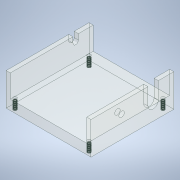
# Autodesk Inventor part: U-shape_v3_0
Saved by Autodesk Inventor 2020 (Build 240168000, 168)
## iProperties
Created: 2022-08-05
Part Number: U-shape_v3_0
Material: Glass
Document SubType Name: Modeling
Designer: Administrator
Density: 2.18 g/cm^3
Appearance: Clear
Author: Administrator
Autodesk Inventor part; units mm, degrees
ref_plane "YZ Plane" through (0, 0, 0) normal (1, 0, 0) x (0, 1, 0)
ref_plane "XZ Plane" through (0, 0, 0) normal (0, 1, 0) x (-1, 0, 0)
ref_plane "XY Plane" through (0, 0, 0) normal (0, 0, 1) x (1, 0, 0)
sketch "Sketch1" plane through (0, 0, 0) normal (0, 1, 0) x (-1, 0, 0)
  line L0 (-43, 37) -> (43, 37)
  line L1 (43, 37) -> (43, -37)
  line L2 (43, -37) -> (-43, -37)
  line L3 (-43, -37) -> (-43, 37)
  line L4 (-43, 37) -> (43, -37) construction
  line L5 (43, 37) -> (-43, -37) construction
  point P0 (0, 0)
  dimension "d0" = 86
  dimension "d1" = 74
  constraints: 12 end point, 2 midpoint, 2 parallel, 1 horizontal, 1 perpendicular
  measures "d0" distance of L1.end L2.end
  measures "d1" distance of L0.end L1.end
extrude "Extrusion1" add sketch "Sketch1" along normal blind 33
sketch "Sketch2" plane through (0, 33, 0) normal (0, 1, 0) x (1, 0, 0)
  line L0 (-43, -37) -> (43, -37) projected
  line L1 (38.75, 40) -> (-38.75, 40)
  line L2 (-38.75, 40) -> (-38.75, -40)
  line L3 (-38.75, -40) -> (38.75, -40)
  line L4 (38.75, -40) -> (38.75, 40)
  line L5 (-38.75, 40) -> (38.75, -40)
  line L6 (-38.75, -40) -> (38.75, 40)
  line L7 (0, 0) -> (-3.3933, 0)
  point P0 (38.75, -37)
  point P1 (-38.75, -37)
  dimension "d8" = 77.5
  dimension "d45" = 80
  constraints: 14 end point, 2 horizontal, 2 parallel, 1 midpoint, 1 perpendicular
  measures "d8" distance of L3.end L2.end
  measures "d45" distance of L3.end L1.start
extrude "Extrusion2" cut sketch "Sketch2" against normal blind 23
sketch "Sketch4" plane through (43, 0, 37) normal (1, 0, 0) x (0, 0, -1)
  line L0 (0, 0) -> (53, 0)
  line L1 (0, 0) -> (74, 0) projected
  line L2 (0, 33) -> (74, 33) projected
  arc A0 (47.75, 16) -> (58.25, 16) centre (53, 16) ccw
  line L3 (58.25, 16) -> (58.25, 33)
  line L4 (74, 33) -> (0, 33) projected
  line L5 (47.75, 16) -> (47.75, 33)
  line L6 (47.75, 33) -> (21.05, 33)
  line L7 (74, 33) -> (0, 33) projected
  line L8 (21.05, 33) -> (21.05, 22.1)
  circle A1 centre (21.05, 22.1) radius 2.75
  point P0 (37, 0)
  dimension "d9" = 53
  dimension "d12" = 10.5
  dimension "d13" = 16
  dimension "d42" = 26.7
  dimension "d43" = 10.9
  dimension "d44" = 5.5
  constraints: 10 end point, 4 point on line, 2 centre point, 2 perpendicular, 2 point on circle, 1 coincident, 1 tangent, 1 vertical
  measures "d9" distance of L0.start L0.end
  measures "d12" diameter of A0
  measures "d13" distance from line of L0 A0.centre
  measures "d42" distance of L5.end L6.end
  measures "d43" distance of L6.end L8.end
  measures "d44" diameter of A1
extrude "Extrusion3" cut sketch "Sketch4" against normal blind 5
sketch "Sketch6" plane through (-43, 0, 37) normal (0, 0, 1) x (1, 0, 0)
  line L0 (86, 0) -> (0, 0) projected
  line L1 (0, 33) -> (86, 33) projected
  line L2 (86, 0) -> (86, 33)
  line L3 (86, 33) -> (81.75, 33)
  line L4 (81.75, 33) -> (81.75, 10)
  line L5 (4.25, 33) -> (4.25, 10) projected
  line L6 (81.75, 10) -> (4.25, 10)
  line L7 (4.25, 10) -> (4.25, 33)
  line L8 (0, 0) -> (0, 33) projected
  line L9 (4.25, 33) -> (0, 33)
  line L10 (0, 33) -> (0, 0)
  line L11 (0, 0) -> (86, 0)
  point P0 (43, 0)
  point P1 (77.5, 2)
  constraints: 16 end point, 7 perpendicular, 1 vertical
extrude "Extrusion4" add sketch "Sketch6" along normal blind 10 contours L0 L8 L1 L5 L6 L4 L2
sketch "Sketch7" plane through (0, 0, 0) normal (0, -1, 0) x (1, 0, 0)
  line L0 (-37.5, -31.5) -> (37.5, -31.5)
  line L1 (37.5, -31.5) -> (37.5, 43.5)
  line L2 (37.5, 43.5) -> (-37.5, 43.5)
  line L3 (-37.5, 43.5) -> (-37.5, -31.5)
  line L4 (-37.5, -31.5) -> (37.5, 43.5) construction
  line L5 (37.5, -31.5) -> (-37.5, 43.5) construction
  circle A0 centre (37.5, 43.5) radius 1.675
  circle A1 centre (37.5, -31.5) radius 1.675
  circle A2 centre (-37.5, 43.5) radius 1.675
  circle A3 centre (-37.5, -31.5) radius 1.675
  point P0 (0, 0)
  dimension "d20" = 75
  dimension "d21" = 75
  dimension "d23" = 3.35
  dimension "d26" = 75
  dimension "d29" = 75
  constraints: 12 end point, 4 centre point, 2 horizontal, 2 parallel, 1 coincident, 1 perpendicular, 1 vertical, 6 other
  measures "d20" distance of L2.end L1.end
  measures "d21" distance of L1.end L0.end
  measures "d23" diameter of A0
  measures "d26" distance of A0.centre A1.centre
  measures "d29" distance of A0.centre A2.centre
extrude "Extrusion5" cut sketch "Sketch7" against normal blind 10 contours L3 A3 L0 | L0 A3 L3 | A1 L1 L0 | L0 L1 A1 | A2 L2 L3 | L3 L2 A2 | A0 L2 L1 | L1 L2 A0
thread "Thread1" size "M3x0.5" class "6H" standard "ANSI Metric M Profile" full length
thread "Thread2" size "M3x0.5" class "6H" standard "ANSI Metric M Profile" full length
thread "Thread3" size "M3x0.5" class "6H" standard "ANSI Metric M Profile" full length
thread "Thread4" size "M3x0.5" class "6H" standard "ANSI Metric M Profile" full length
sketch "Sketch8" plane through (-43, 0, -37) normal (-1, 0, 0) x (0, 0, 1)
  line L0 (84, 10) -> (0, 10) projected
  line L1 (15.75, 10) -> (15.75, 0)
  line L2 (0, 0) -> (84, 0) projected
  line L3 (15.75, 0) -> (17.75, 0)
  line L4 (17.75, 0) -> (17.75, 27.4)
  circle A0 centre (17.75, 27.4) radius 2.75
  line L5 (15.75, 33) -> (15.75, 16) projected
  line L6 (20.5, 27.4) -> (20.5, 33)
  line L7 (15, 27.4) -> (15, 33)
  line L8 (0, 33) -> (84, 33) projected
  point P0 (37, 0)
  point P1 (17.228, 33)
  point P2 (18.272, 33)
  dimension "d46" = 2
  dimension "d47" = 27.4
  dimension "d48" = 5.5
  dimension "d51" = 0
  constraints: 10 end point, 5 point on line, 3 vertical, 2 point on circle, 1 centre point, 1 coincident, 1 perpendicular, 1 tangent
  measures "d46" distance of L1.end L3.end
  measures "d47" distance of L3.end L4.end
  measures "d48" diameter of A0
  measures "d51" distance from line of L5 L1.end
extrude "Extrusion6" cut sketch "Sketch8" against normal blind 10 contours A0 L5 | A0 L5 | A0 L5 L8 L6 | L7 L8 L5 A0
sketch "Sketch10" plane through (37.5, 8, 43.5) normal (1, 0, 0) x (0, 0, 1)
  line L0 (1.675, 0) -> (1.675, 8)
  line L1 (1.675, 8) -> (1.3043, 8)
  line L2 (1.3043, 8) -> (1.3043, 0)
  line L3 (1.3043, 0) -> (1.675, 0)
  line L4 (0, -1.6) -> (0, 9.6) projected
  constraints: 8 end point
revolve "Revolution1" add sketch "Sketch10" angle 360 about axis through (37.5, 8, 43.5) along (0, -1, 0) separate body
sketch "Sketch9" plane through (37.5, 8, 45.175) normal (-1, 0, 0) x (0, -1, 0)
  line L0 (-0.2918, -0.0255) -> (-0.2501, -0.0255) construction
  line L1 (0.0416, -0.3456) -> (-0.0001, -0.4257) construction
  line L2 (-0.5001, -0.4257) -> (-0.5418, -0.3456) construction
  line L3 (-0.2084, -0.0255) -> (-0.2501, 0.0546) construction
  line L4 (-0.2501, 0.0546) -> (-0.2918, -0.0255) construction
  line L5 (-0.5001, -0.4257) -> (-0.4584, -0.3456) construction
  line L6 (-0.2084, -0.0255) -> (-0.0418, -0.3456)
  line L7 (-0.5418, -0.3456) -> (-0.4584, -0.3456) construction
  arc A0 (-0.5418, -0.3456) -> (-0.5001, -0.3709) centre (-0.5001, -0.3239) ccw construction
  line L8 (0.0416, -0.3456) -> (-0.0418, -0.3456) construction
  line L9 (-0.5001, -0.4257) -> (-0.5001, -0.3456) construction
  line L10 (-0.0001, -0.4257) -> (-0.0001, -0.3456) construction
  line L11 (-0.2501, 0.0546) -> (-0.2501, -0.0002) construction
  line L12 (-0.5001, -0.3709) -> (-0.0001, -0.3709)
  arc A1 (-0.5001, -0.3709) -> (-0.4584, -0.3456) centre (-0.5001, -0.3239) ccw
  line L13 (-0.0418, -0.3456) -> (-0.0001, -0.4257) construction
  line L14 (-0.4584, -0.3456) -> (-0.2918, -0.0255)
  line L15 (-0.0001, -0.0002) -> (-0.0001, 0.0177)
  line L16 (-0.0001, 0.0177) -> (-0.0001, -0.0002)
  line L17 (-0.0001, -0.0002) -> (0.0334, -0.0002)
  arc A2 (-0.0418, -0.3456) -> (-0.0001, -0.3709) centre (-0.0001, -0.3239) ccw
  arc A3 (-0.0001, -0.3709) -> (0.0416, -0.3456) centre (-0.0001, -0.3239) ccw construction
  arc A4 (-0.2501, -0.0002) -> (-0.2918, -0.0255) centre (-0.2501, -0.0471) ccw
  arc A5 (-0.2084, -0.0255) -> (-0.2501, -0.0002) centre (-0.2501, -0.0471) ccw
  line L18 (-0.2501, -0.0002) -> (-0.2501, -0.0255) construction
  line L19 (-0.2501, -0.0255) -> (-0.2084, -0.0255) construction
  dimension "d52" = 55
  dimension "d53" = 0.08
  dimension "d54" = 0.08
  dimension "Sketch9_ThreadOffset" = 0
  dimension "Sketch9_MajorRadius" = 0.3707
  dimension "d57" = 0.5
  dimension "Sketch9_MinorRadius" = 0
  constraints: 40 end point, 12 point on circle, 10 parallel, 8 tangent, 6 centre point, 6 collinear, 2 midpoint, 2 point on line, 1 horizontal, 1 perpendicular, 3 other
  measures "d52" angle of L6 L14
  measures "d53" distance of L3.end L0.end
  measures "d54" distance of L1.end L10.end
  measures "Sketch9_ThreadOffset" distance between parallel lines of L15 L10
  measures "Sketch9_MajorRadius" distance from line of L12 L15.start
  measures "d57" distance from line of L1.end L9
  measures "Sketch9_MinorRadius" distance edge to line of A5 L17
coil "Coil1" sketch "Sketch9" operation cut axis through (37.5, 8, 43.5) along (0, -1, 0) pitch 0.5005 turns 17.982018 hand right bodies 2
sketch "Sketch12" plane through (-37.5, 8, 43.5) normal (1, 0, 0) x (0, 0, 1)
  line L0 (1.675, 0) -> (1.675, 8)
  line L1 (1.675, 8) -> (1.3043, 8)
  line L2 (1.3043, 8) -> (1.3043, 0)
  line L3 (1.3043, 0) -> (1.675, 0)
  line L4 (0, -1.6) -> (0, 9.6) projected
  constraints: 8 end point
revolve "Revolution2" add sketch "Sketch12" angle 360 about axis through (-37.5, 8, 43.5) along (0, -1, 0) separate body
sketch "Sketch11" plane through (-37.5, 8, 45.175) normal (-1, 0, 0) x (0, -1, 0)
  line L0 (-0.2918, -0.0255) -> (-0.2501, -0.0255) construction
  line L1 (0.0416, -0.3456) -> (-0.0001, -0.4257) construction
  line L2 (-0.5001, -0.4257) -> (-0.5418, -0.3456) construction
  line L3 (-0.2084, -0.0255) -> (-0.2501, 0.0546) construction
  line L4 (-0.2501, 0.0546) -> (-0.2918, -0.0255) construction
  line L5 (-0.5001, -0.4257) -> (-0.4584, -0.3456) construction
  line L6 (-0.2084, -0.0255) -> (-0.0418, -0.3456)
  line L7 (-0.5418, -0.3456) -> (-0.4584, -0.3456) construction
  arc A0 (-0.5418, -0.3456) -> (-0.5001, -0.3709) centre (-0.5001, -0.3239) ccw construction
  line L8 (0.0416, -0.3456) -> (-0.0418, -0.3456) construction
  line L9 (-0.5001, -0.4257) -> (-0.5001, -0.3456) construction
  line L10 (-0.0001, -0.4257) -> (-0.0001, -0.3456) construction
  line L11 (-0.2501, 0.0546) -> (-0.2501, -0.0002) construction
  line L12 (-0.5001, -0.3709) -> (-0.0001, -0.3709)
  arc A1 (-0.5001, -0.3709) -> (-0.4584, -0.3456) centre (-0.5001, -0.3239) ccw
  line L13 (-0.0418, -0.3456) -> (-0.0001, -0.4257) construction
  line L14 (-0.4584, -0.3456) -> (-0.2918, -0.0255)
  line L15 (-0.0001, -0.0002) -> (-0.0001, 0.0177)
  line L16 (-0.0001, 0.0177) -> (-0.0001, -0.0002)
  line L17 (-0.0001, -0.0002) -> (0.0334, -0.0002)
  arc A2 (-0.0418, -0.3456) -> (-0.0001, -0.3709) centre (-0.0001, -0.3239) ccw
  arc A3 (-0.0001, -0.3709) -> (0.0416, -0.3456) centre (-0.0001, -0.3239) ccw construction
  arc A4 (-0.2501, -0.0002) -> (-0.2918, -0.0255) centre (-0.2501, -0.0471) ccw
  arc A5 (-0.2084, -0.0255) -> (-0.2501, -0.0002) centre (-0.2501, -0.0471) ccw
  line L18 (-0.2501, -0.0002) -> (-0.2501, -0.0255) construction
  line L19 (-0.2501, -0.0255) -> (-0.2084, -0.0255) construction
  dimension "d70" = 55
  dimension "d71" = 0.08
  dimension "d72" = 0.08
  dimension "Sketch11_ThreadOffset" = 0
  dimension "Sketch11_MajorRadius" = 0.3707
  dimension "d75" = 0.5
  dimension "Sketch11_MinorRadius" = 0
  constraints: 40 end point, 12 point on circle, 10 parallel, 8 tangent, 6 centre point, 6 collinear, 2 midpoint, 2 point on line, 1 horizontal, 1 perpendicular, 3 other
  measures "d70" angle of L6 L14
  measures "d71" distance of L3.end L0.end
  measures "d72" distance of L1.end L10.end
  measures "Sketch11_ThreadOffset" distance between parallel lines of L15 L10
  measures "Sketch11_MajorRadius" distance from line of L12 L15.start
  measures "d75" distance from line of L1.end L9
  measures "Sketch11_MinorRadius" distance edge to line of A5 L17
coil "Coil2" sketch "Sketch11" operation cut axis through (-37.5, 8, 43.5) along (0, -1, 0) pitch 0.5005 turns 17.982018 hand right bodies 3
sketch "Sketch14" plane through (37.5, 8, -31.5) normal (1, 0, 0) x (0, 0, 1)
  line L0 (1.675, 0) -> (1.675, 8)
  line L1 (1.675, 8) -> (1.3043, 8)
  line L2 (1.3043, 8) -> (1.3043, 0)
  line L3 (1.3043, 0) -> (1.675, 0)
  line L4 (0, -1.6) -> (0, 9.6) projected
  constraints: 8 end point
revolve "Revolution3" add sketch "Sketch14" angle 360 about axis through (37.5, 8, -31.5) along (0, -1, 0) separate body
sketch "Sketch13" plane through (37.5, 8, -29.825) normal (-1, 0, 0) x (0, -1, 0)
  line L0 (-0.2918, -0.0255) -> (-0.2501, -0.0255) construction
  line L1 (0.0416, -0.3456) -> (-0.0001, -0.4257) construction
  line L2 (-0.5001, -0.4257) -> (-0.5418, -0.3456) construction
  line L3 (-0.2084, -0.0255) -> (-0.2501, 0.0546) construction
  line L4 (-0.2501, 0.0546) -> (-0.2918, -0.0255) construction
  line L5 (-0.5001, -0.4257) -> (-0.4584, -0.3456) construction
  line L6 (-0.2084, -0.0255) -> (-0.0418, -0.3456)
  line L7 (-0.5418, -0.3456) -> (-0.4584, -0.3456) construction
  arc A0 (-0.5418, -0.3456) -> (-0.5001, -0.3709) centre (-0.5001, -0.3239) ccw construction
  line L8 (0.0416, -0.3456) -> (-0.0418, -0.3456) construction
  line L9 (-0.5001, -0.4257) -> (-0.5001, -0.3456) construction
  line L10 (-0.0001, -0.4257) -> (-0.0001, -0.3456) construction
  line L11 (-0.2501, 0.0546) -> (-0.2501, -0.0002) construction
  line L12 (-0.5001, -0.3709) -> (-0.0001, -0.3709)
  arc A1 (-0.5001, -0.3709) -> (-0.4584, -0.3456) centre (-0.5001, -0.3239) ccw
  line L13 (-0.0418, -0.3456) -> (-0.0001, -0.4257) construction
  line L14 (-0.4584, -0.3456) -> (-0.2918, -0.0255)
  line L15 (-0.0001, -0.0002) -> (-0.0001, 0.0177)
  line L16 (-0.0001, 0.0177) -> (-0.0001, -0.0002)
  line L17 (-0.0001, -0.0002) -> (0.0334, -0.0002)
  arc A2 (-0.0418, -0.3456) -> (-0.0001, -0.3709) centre (-0.0001, -0.3239) ccw
  arc A3 (-0.0001, -0.3709) -> (0.0416, -0.3456) centre (-0.0001, -0.3239) ccw construction
  arc A4 (-0.2501, -0.0002) -> (-0.2918, -0.0255) centre (-0.2501, -0.0471) ccw
  arc A5 (-0.2084, -0.0255) -> (-0.2501, -0.0002) centre (-0.2501, -0.0471) ccw
  line L18 (-0.2501, -0.0002) -> (-0.2501, -0.0255) construction
  line L19 (-0.2501, -0.0255) -> (-0.2084, -0.0255) construction
  dimension "d88" = 55
  dimension "d89" = 0.08
  dimension "d90" = 0.08
  dimension "Sketch13_ThreadOffset" = 0
  dimension "Sketch13_MajorRadius" = 0.3707
  dimension "d93" = 0.5
  dimension "Sketch13_MinorRadius" = 0
  constraints: 40 end point, 12 point on circle, 10 parallel, 8 tangent, 6 centre point, 6 collinear, 2 midpoint, 2 point on line, 1 horizontal, 1 perpendicular, 3 other
  measures "d88" angle of L6 L14
  measures "d89" distance of L3.end L0.end
  measures "d90" distance of L1.end L10.end
  measures "Sketch13_ThreadOffset" distance between parallel lines of L15 L10
  measures "Sketch13_MajorRadius" distance from line of L12 L15.start
  measures "d93" distance from line of L1.end L9
  measures "Sketch13_MinorRadius" distance edge to line of A5 L17
coil "Coil3" sketch "Sketch13" operation cut axis through (37.5, 8, -31.5) along (0, -1, 0) pitch 0.5005 turns 17.982018 hand right bodies 4
sketch "Sketch16" plane through (-37.5, 8, -31.5) normal (1, 0, 0) x (0, 0, 1)
  line L0 (1.675, 0) -> (1.675, 8)
  line L1 (1.675, 8) -> (1.3043, 8)
  line L2 (1.3043, 8) -> (1.3043, 0)
  line L3 (1.3043, 0) -> (1.675, 0)
  line L4 (0, -1.6) -> (0, 9.6) projected
  constraints: 8 end point
revolve "Revolution4" add sketch "Sketch16" angle 360 about axis through (-37.5, 8, -31.5) along (0, -1, 0) separate body
sketch "Sketch15" plane through (-37.5, 8, -29.825) normal (-1, 0, 0) x (0, -1, 0)
  line L0 (-0.2918, -0.0255) -> (-0.2501, -0.0255) construction
  line L1 (0.0416, -0.3456) -> (-0.0001, -0.4257) construction
  line L2 (-0.5001, -0.4257) -> (-0.5418, -0.3456) construction
  line L3 (-0.2084, -0.0255) -> (-0.2501, 0.0546) construction
  line L4 (-0.2501, 0.0546) -> (-0.2918, -0.0255) construction
  line L5 (-0.5001, -0.4257) -> (-0.4584, -0.3456) construction
  line L6 (-0.2084, -0.0255) -> (-0.0418, -0.3456)
  line L7 (-0.5418, -0.3456) -> (-0.4584, -0.3456) construction
  arc A0 (-0.5418, -0.3456) -> (-0.5001, -0.3709) centre (-0.5001, -0.3239) ccw construction
  line L8 (0.0416, -0.3456) -> (-0.0418, -0.3456) construction
  line L9 (-0.5001, -0.4257) -> (-0.5001, -0.3456) construction
  line L10 (-0.0001, -0.4257) -> (-0.0001, -0.3456) construction
  line L11 (-0.2501, 0.0546) -> (-0.2501, -0.0002) construction
  line L12 (-0.5001, -0.3709) -> (-0.0001, -0.3709)
  arc A1 (-0.5001, -0.3709) -> (-0.4584, -0.3456) centre (-0.5001, -0.3239) ccw
  line L13 (-0.0418, -0.3456) -> (-0.0001, -0.4257) construction
  line L14 (-0.4584, -0.3456) -> (-0.2918, -0.0255)
  line L15 (-0.0001, -0.0002) -> (-0.0001, 0.0177)
  line L16 (-0.0001, 0.0177) -> (-0.0001, -0.0002)
  line L17 (-0.0001, -0.0002) -> (0.0334, -0.0002)
  arc A2 (-0.0418, -0.3456) -> (-0.0001, -0.3709) centre (-0.0001, -0.3239) ccw
  arc A3 (-0.0001, -0.3709) -> (0.0416, -0.3456) centre (-0.0001, -0.3239) ccw construction
  arc A4 (-0.2501, -0.0002) -> (-0.2918, -0.0255) centre (-0.2501, -0.0471) ccw
  arc A5 (-0.2084, -0.0255) -> (-0.2501, -0.0002) centre (-0.2501, -0.0471) ccw
  line L18 (-0.2501, -0.0002) -> (-0.2501, -0.0255) construction
  line L19 (-0.2501, -0.0255) -> (-0.2084, -0.0255) construction
  dimension "d106" = 55
  dimension "d107" = 0.08
  dimension "d108" = 0.08
  dimension "Sketch15_ThreadOffset" = 0
  dimension "Sketch15_MajorRadius" = 0.3707
  dimension "d111" = 0.5
  dimension "Sketch15_MinorRadius" = 0
  constraints: 40 end point, 12 point on circle, 10 parallel, 8 tangent, 6 centre point, 6 collinear, 2 midpoint, 2 point on line, 1 horizontal, 1 perpendicular, 3 other
  measures "d106" angle of L6 L14
  measures "d107" distance of L3.end L0.end
  measures "d108" distance of L1.end L10.end
  measures "Sketch15_ThreadOffset" distance between parallel lines of L15 L10
  measures "Sketch15_MajorRadius" distance from line of L12 L15.start
  measures "d111" distance from line of L1.end L9
  measures "Sketch15_MinorRadius" distance edge to line of A5 L17
coil "Coil4" sketch "Sketch15" operation cut axis through (-37.5, 8, -31.5) along (0, -1, 0) pitch 0.5005 turns 17.982018 hand right bodies 5
equation "\"d52\" = d59"
equation "\"d53\" = 0.160083 * Sketch9_Pitch"
equation "\"d54\" = 0.160083 * Sketch9_Pitch"
equation "\"d57\" = Sketch9_Pitch"
equation "\"d70\" = d77"
equation "\"d71\" = 0.160083 * Sketch11_Pitch"
equation "\"d72\" = 0.160083 * Sketch11_Pitch"
equation "\"d75\" = Sketch11_Pitch"
equation "\"d88\" = d95"
equation "\"d89\" = 0.160083 * Sketch13_Pitch"
equation "\"d90\" = 0.160083 * Sketch13_Pitch"
equation "\"d93\" = Sketch13_Pitch"
equation "\"d106\" = d113"
equation "\"d107\" = 0.160083 * Sketch15_Pitch"
equation "\"d108\" = 0.160083 * Sketch15_Pitch"
equation "\"d111\" = Sketch15_Pitch"
equation "\"d59\" = 55deg"
equation "\"Sketch9_Pitch\" = 0.5"
equation "\"d77\" = 55deg"
equation "\"Sketch11_Pitch\" = 0.5"
equation "\"d95\" = 55deg"
equation "\"Sketch13_Pitch\" = 0.5"
equation "\"d113\" = 55deg"
equation "\"Sketch15_Pitch\" = 0.5"
body "Solid1"
body "Solid2"
body "Solid3"
body "Solid4"
body "Solid5"
